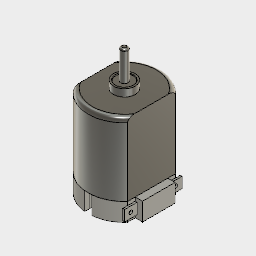
711 DC Toy Motor (Autodesk Fusion 360 design; units mm, degrees)
Autodesk Fusion 360 part; units mm, degrees
note: some values were not read from the file. Set by a fixed rule: which sketch regions a step uses.
sketch "Sketch1" plane through (0, 0, 0) normal (0, 0, 1) x (1, 0, 0)
  line L0 (7.5, -10) -> (-7.5, -10)
  line L1 (-7.5, -10) -> (-7.5, 10)
  line L2 (-7.5, 10) -> (7.5, 10)
  line L3 (7.5, 10) -> (7.5, -10)
  line L4 (7.5, -10) -> (-7.5, 10) construction
  line L5 (-7.5, -10) -> (7.5, 10) construction
  circle A0 centre (0, 0) radius 10
  dimension "d1" = 15
  dimension "d2" = 20
  dimension "d3" = 20
  measures "d1" distance of L1.end L2.end
  measures "d2" distance of L0.end L1.end
  measures "d3" diameter of A0
extrude "Extrude1" add sketch "Sketch1" along normal blind 20 contours L1 L3 A0 makes body 1
sketch "Sketch2" plane through (0, 0, 20) normal (0, 0, 1) x (-1, 0, 0)
  arc A0 (7.5, 6.6144) -> (-7.5, 6.6144) centre (0, 0) ccw
  line L0 (-7.5, 6.6144) -> (-7.5, -6.6144)
  arc A1 (-7.5, -6.6144) -> (7.5, -6.6144) centre (0, 0) ccw
  line L1 (7.5, -6.6144) -> (7.5, 6.6144)
  circle A2 centre (0, 0) radius 3
  circle A3 centre (0, 0) radius 1
  circle A4 centre (0, 0) radius 2.5
  circle A5 centre (0, 0) radius 2.4
  dimension "d6" = 6
  dimension "d7" = 2
  dimension "d8" = 0.5
  dimension "d14" = 0.1
  measures "d6" diameter of A2
  measures "d7" diameter of A3
  measures "d14" distance of A4 A5
extrude "Extrude2" add sketch "Sketch2" along normal blind 2 contours A2 bodies 1
extrude "Extrude3" add sketch "Sketch2" along normal blind 10 contours A3 bodies 1
fillet "Fillet1" radius 0.5 1 edges at (0.9323, 0.3616, 30) on bodies 1
extrude "Extrude4" add sketch "Sketch2" along normal blind 1.8 contours A5 bodies 1
fillet "Fillet2" radius 1.2 2 edges at (0, -10, 20) (0, 10, 20) on bodies 1
sketch "Sketch3" plane through (0, 0, 0) normal (0, 0, -1) x (1, 0, 0)
  arc A0 (7.5, 6.6144) -> (-7.5, 6.6144) centre (0, 0) ccw
  line L0 (-7.5, 6.6144) -> (-7.5, -6.6144)
  arc A1 (-7.5, -6.6144) -> (7.5, -6.6144) centre (0, 0) ccw
  line L1 (7.5, -6.6144) -> (7.5, 6.6144)
  line L2 (-1, -10) -> (1, -10)
  line L3 (1, -10) -> (1, -7.5)
  line L4 (1, -7.5) -> (-1, -7.5)
  line L5 (-1, -7.5) -> (-1, -10)
  line L6 (0, 0) -> (-7.5, 0) construction
  line L7 (1, 10) -> (1, 7.5)
  line L8 (1, 7.5) -> (-1, 7.5)
  line L9 (-1, 7.5) -> (-1, 10)
  line L10 (-1, 10) -> (1, 10)
  line L11 (9.5, -4.5) -> (7.5, -4.5)
  line L12 (7.5, -4.5) -> (7.5, 4.5)
  line L13 (7.5, 4.5) -> (9.5, 4.5)
  line L14 (9.5, 4.5) -> (9.5, -4.5)
  line L15 (9.5, -4.5) -> (7.5, 4.5) construction
  line L16 (7.5, -4.5) -> (9.5, 4.5) construction
  point P0 (8.5, 0)
  dimension "d18" = 2.5
  dimension "d22" = 9
  dimension "d23" = 2
  measures "d18" distance of L2.start L4.end
  measures "d22" distance of L11.end L12.end
  measures "d23" distance of L12.end L13.end
extrude "Extrude5" add sketch "Sketch3" along normal blind 5 separate body contours A0 L0 A1 L1 L3 L4 L5 L7 L8 L9 L12 | L1 L11 L12 L13 L14 makes body 2
fillet "Fillet3" radius 1 4 edges at (1, -7.5, -2.5) (-1, -7.5, -2.5) (1, 7.5, -2.5) (-1, 7.5, -2.5) on bodies 2
sketch "Sketch4" plane through (0, 0, -5) normal (0, 0, -1) x (1, 0, 0)
  line L0 (7.5, 4.5) -> (7.5, 6.6144)
  arc A0 (7.5, 6.6144) -> (1, 9.9499) centre (0, 0) ccw
  line L1 (1, 9.9499) -> (1, 8.5)
  arc A1 (0, 7.5) -> (1, 8.5) centre (0, 8.5) ccw
  arc A2 (-1, 8.5) -> (0, 7.5) centre (0, 8.5) ccw
  line L2 (-1, 8.5) -> (-1, 9.9499)
  arc A3 (-1, 9.9499) -> (-7.5, 6.6144) centre (0, 0) ccw
  line L3 (-7.5, 6.6144) -> (-7.5, -6.6144)
  arc A4 (-7.5, -6.6144) -> (-1, -9.9499) centre (0, 0) ccw
  line L4 (-1, -9.9499) -> (-1, -8.5)
  arc A5 (0, -7.5) -> (-1, -8.5) centre (0, -8.5) ccw
  arc A6 (1, -8.5) -> (0, -7.5) centre (0, -8.5) ccw
  line L5 (1, -8.5) -> (1, -9.9499)
  arc A7 (1, -9.9499) -> (7.5, -6.6144) centre (0, 0) ccw
  line L6 (7.5, -6.6144) -> (7.5, -4.5)
  line L7 (7.5, -4.5) -> (9.5, -4.5)
  line L8 (9.5, -4.5) -> (9.5, 4.5)
  line L9 (9.5, 4.5) -> (7.5, 4.5)
  circle A8 centre (0, 0) radius 4.9
  line L10 (-4, 5.5) -> (-4, -5.5)
  dimension "d24" = 9.8
  dimension "d26" = 4
  measures "d24" diameter of A8
  measures "d26" distance of A0.centre L10
extrude "Extrude6" add sketch "Sketch4" along normal blind 2 contours A8 L10 picked at (-0.1396, 1.4091) bodies 2
sketch "Sketch5" plane through (0, 0, -7) normal (0, 0, -1) x (1, 0, 0)
  arc A0 (-4, -2.8302) -> (-4, 2.8302) centre (0, 0) ccw
  line L0 (-4, 2.8302) -> (-4, -2.8302)
  circle A1 centre (0, 0) radius 1
  line L1 (2.5, -2.5) -> (3.5, -2.5)
  line L2 (3.5, -2.5) -> (3.5, 2.5)
  line L3 (3.5, 2.5) -> (2.5, 2.5)
  line L4 (2.5, 2.5) -> (2.5, -2.5)
  line L5 (2.5, -2.5) -> (3.5, 2.5) construction
  line L6 (3.5, -2.5) -> (2.5, 2.5) construction
  line L7 (3, 0) -> (0, 0) construction
  point P0 (3, 0)
  dimension "d29" = 2
  dimension "d33" = 1
  dimension "d34" = 5
  dimension "d35" = 3
  measures "d29" diameter of A1
  measures "d33" distance of L2.end L3.end
  measures "d34" distance of L1.end L2.end
  measures "d35" distance of A0.centre P0
extrude "Extrude8" cut sketch "Sketch5" against normal blind 2 contours L1 L2 L3 L4 bodies 2
extrude "Extrude7" add sketch "Sketch5" along normal blind 1 contours A1 bodies 2
fillet "Fillet4" radius 0.5 1 edges at (-0.9323, 0.3616, -8) on bodies 2
sketch "Sketch6" plane through (7.5, 0, 0) normal (1, 0, 0) x (0, 1, 0)
  line L0 (-4.5, 0) -> (-6.6144, 0)
  line L1 (-6.6144, 0) -> (-6.6144, -5) construction
  line L2 (-6.6144, -5) -> (-4.5, -5)
  line L3 (-4.5, -5) -> (-4.5, 0)
  line L4 (6.6144, 0) -> (4.5, 0)
  line L5 (4.5, 0) -> (4.5, -5)
  line L6 (4.5, -5) -> (6.6144, -5)
  line L7 (6.6144, -5) -> (6.6144, 0) construction
  line L8 (-4.5, -1) -> (-7.9499, -1)
  line L9 (-7.9499, -1) -> (-7.9499, -4)
  line L10 (-7.9499, -4) -> (-4.5, -4)
  line L11 (-4.5, -4) -> (-4.5, -1)
  line L12 (-9.9499, 0) -> (-9.9499, -5)
  line L13 (-9.9499, 0) -> (-6.6144, 0)
  line L14 (-9.9499, -5) -> (-6.6144, -5)
  line L15 (4.5, -5) -> (-4.5, -5)
  line L16 (0, 0) -> (0, -5) construction
  line L17 (7.9499, -4) -> (4.5, -4)
  line L18 (4.5, -4) -> (4.5, -1)
  line L19 (4.5, -1) -> (7.9499, -1)
  line L20 (7.9499, -1) -> (7.9499, -4)
  circle A0 centre (-6.2249, -2.5) radius 0.5
  circle A1 centre (6.2249, -2.5) radius 0.5
  dimension "d38" = 1
  dimension "d39" = 1
  dimension "d42" = 2
  dimension "d43" = 1
  measures "d38" distance of L8 L13
  measures "d39" distance of L10 L14
  measures "d42" distance of L9 L12
  measures "d43" diameter of A0
extrude "Extrude9" add sketch "Sketch6" along normal blind 0.5 contours L3 L8 L9 L10 L11 | L5 L17 L18 L19 L20 bodies 2
